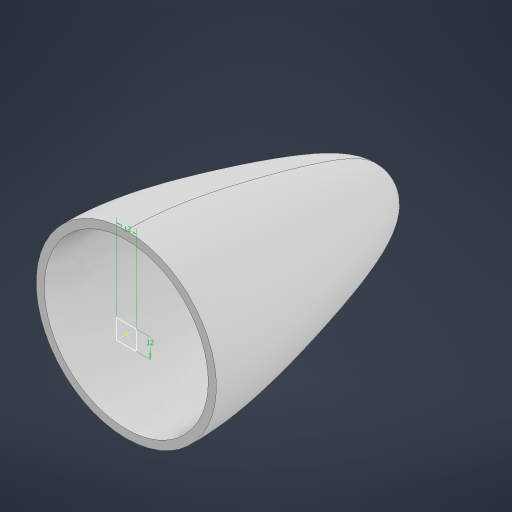
# Autodesk Inventor part: WKA CAD
Saved by Autodesk Inventor 2023.2 (Build 272271000, 271)
## iProperties
Created: 2022-12-22
Part Number: WKA CAD
Material: Generisch
Document SubType Name: Modeling
Designer: tadeu
Density: 1 g/cm^3
Appearance: Vorgabe
Author: tadeu
Autodesk Inventor part; units mm, degrees
ref_plane "YZ Plane" through (0, 0, 0) normal (1, 0, 0) x (0, 1, 0)
ref_plane "XZ Plane" through (0, 0, 0) normal (0, 1, 0) x (-1, 0, 0)
ref_plane "XY Plane" through (0, 0, 0) normal (0, 0, 1) x (1, 0, 0)
sketch "Skizze4" plane through (0, 0, 0) normal (1, 0, 0) x (0, 1, 0)
  line L0 (0, 0) -> (0, 80)
  line L1 (0, 0) -> (0, -160)
  line L2 (0, 80) -> (40.0393, 78.1112) construction
  line L3 (40.0393, 78.1112) -> (79.6393, 0) construction
  line L4 (79.6393, 0) -> (35.7633, -87.3536) construction
  line L5 (35.7633, -87.3536) -> (24.8721, -160) construction
  line L6 (24.8721, -160) -> (0, -160) construction
  spline S0 degree 4 poles (0, 80) (40.0393, 78.1112) (79.6393, 0) (35.7633, -87.3536) (24.8721, -160) (0, -160) knots 1 1 1 1 1 2 3 3 3 3 3
  line L7 (0, 0) -> (55.5455, 0)
  dimension "d2" = 80
  dimension "d3" = 160
  constraints: 6 end point, 2 vertical, 1 horizontal, 4 other
  measures "d2" distance of L0.start L0.end
  measures "d3" distance of L0.start L1.end
revolve "Umdrehung1" add sketch "Skizze4" angle 360 about axis through (0, 0, 0) along (0, 0, 1) contours L0 S0 L7
revolve "Umdrehung2" add sketch "Skizze4" angle 360 about axis through (0, 0, 0) along (0, 0, -1) separate body contours L7 S0 L1
move or copy body "Körper verschieben1" bodies to move or copy 1 copy no translate (0, 0, 50)
shell "Wandung3" thickness 5 removed faces 2 at (-14.7754, -16.2079, 50) at (6.6884, -0.759, 0) bodies 1 2
sketch "Skizze10" plane through (0, 0, 0) normal (0, 0, 1) x (1, 0, 0)
  line L0 (-6, 6) -> (6, 6)
  line L1 (6, 6) -> (6, -6)
  line L2 (6, -6) -> (-6, -6)
  line L3 (-6, -6) -> (-6, 6)
  line L4 (-6, 6) -> (6, -6) construction
  line L5 (6, 6) -> (-6, -6) construction
  point P0 (0, 0)
  dimension "d22" = 12
  dimension "d23" = 12
  constraints: 12 end point, 2 midpoint, 2 parallel, 1 horizontal, 1 perpendicular
  measures "d22" distance of L0.start L0.end
  measures "d23" distance of L0.end L1.end
